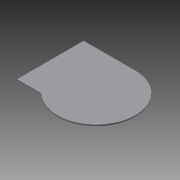
# Autodesk Inventor part: Base_Right
Saved by Autodesk Inventor 2014 SP1 (Build 180222100, 222)
## iProperties
Created: 2014-01-12
Part Number: Base_Right
Material: Generic
Document SubType Name: Modeling
Designer: tuleu
Density: 1 g/cm^3
Appearance: Default
Author: tuleu
Autodesk Inventor part; units mm, degrees
ref_plane "YZ Plane" through (0, 0, 0) normal (1, 0, 0) x (0, 1, 0)
ref_plane "XZ Plane" through (0, 0, 0) normal (0, 1, 0) x (-1, 0, 0)
ref_plane "XY Plane" through (0, 0, 0) normal (0, 0, 1) x (1, 0, 0)
sketch "Sketch1" plane through (0, 0, 0) normal (0, 1, 0) x (-1, 0, 0)
  arc A0 (342.9286, 350) -> (0, -490) centre (0, 0) ccw
  line L0 (0, -490) -> (650, -490)
  line L1 (650, -490) -> (650, 350)
  line L2 (650, 350) -> (342.9286, 350)
  dimension "d0" = 490
  dimension "d1" = 650
  dimension "d2" = 350
  constraints: 6 end point, 2 point on circle, 1 centre point, 1 coincident, 1 horizontal, 1 parallel, 1 perpendicular, 1 tangent
  measures "d0" radius of A0
  measures "d1" distance from line of point (0, 0) L1
  measures "d2" distance from line of point (0, 0) L2
extrude "Extrusion1" add sketch "Sketch1" along normal mid plane 16
body "Solid1"
